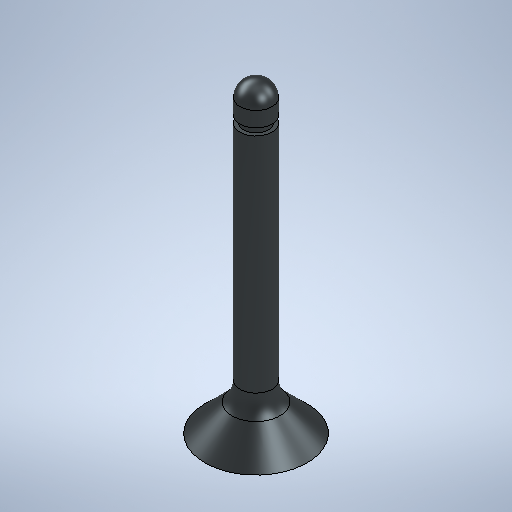
# Autodesk Inventor part: Ventil
Saved by Autodesk Inventor 2025 (Build 290162010, 162A)
## iProperties
Created: 2024-07-15
Part Number: Ventil
Material: Iron, Gray
Document SubType Name: Modeling
Designer: Fabri
Density: 7.15 g/cm^3
Appearance: Iron Gray
Author: Fabri
Autodesk Inventor part; units mm, degrees
ref_plane "YZ Plane" through (0, 0, 0) normal (1, 0, 0) x (0, 1, 0)
ref_plane "XZ Plane" through (0, 0, 0) normal (0, 1, 0) x (-1, 0, 0)
ref_plane "XY Plane" through (0, 0, 0) normal (0, 0, 1) x (1, 0, 0)
sketch "Sketch1" plane through (0, 0, 0) normal (0, 1, 0) x (-1, 0, 0)
  line L0 (0, 0) -> (4.75, 0)
  line L1 (4.75, 0) -> (1.5, 3.25)
  line L2 (1.5, 3.25) -> (1.5, 24.95)
  line L3 (1.5, 24.95) -> (1.15, 24.95)
  line L4 (1.15, 24.95) -> (1.15, 25.6)
  line L5 (1.15, 25.6) -> (1.5, 25.6)
  line L6 (1.5, 25.6) -> (1.5, 27)
  arc A0 (1.5, 27) -> (0, 28.5) centre (0, 27) ccw
  line L7 (0, 28.5) -> (0, 0)
  point P0 (0, 14.25)
  dimension "d4" = 45
  dimension "d5" = 9.5
  dimension "d6" = 3
  dimension "d7" = 0.65
  dimension "d8" = 2.3
  dimension "d9" = 2.9
  dimension "d10" = 28.5
  constraints: 16 end point, 4 perpendicular, 3 point on line, 2 point on circle, 1 centre point, 1 horizontal, 1 midpoint, 1 tangent, 1 vertical
  measures "d4" angle of L0 L1
  measures "d5" diameter of L0.end L7
  measures "d6" diameter of L2 point (0, 14.25)
  measures "d7" distance of L3.end L4.end
  measures "d8" diameter of L4 L7
  measures "d9" vertical distance of L7.start L4.end
  measures "d10" distance of L0.start L7.start
revolve "Revolution1" add sketch "Sketch1" angle 360 about axis through (0, 0, 28.5) along (0, 0, -1)
fillet "Fillet1" radius 2.5 1 edges at (1.5, 0, 3.25)
body "Solid1"
